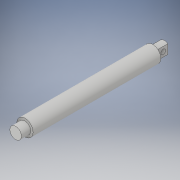
# Autodesk Inventor part: 4in stroke cylinder
Saved by Autodesk Inventor 2017 (Build 210142000, 142)
## iProperties
Created: 2017-01-19
Part Number: 4in stroke cylinder
Material: Generic
Document SubType Name: Modeling
Designer: Ben
Density: 1 g/cm^3
Appearance: Default
Author: Ben
Autodesk Inventor part; units mm, degrees
ref_plane "YZ Plane" through (0, 0, 0) normal (1, 0, 0) x (0, 1, 0)
ref_plane "XZ Plane" through (0, 0, 0) normal (0, 1, 0) x (-1, 0, 0)
ref_plane "XY Plane" through (0, 0, 0) normal (0, 0, 1) x (1, 0, 0)
sketch "Sketch1" plane through (0, 0, 0) normal (0, 0, 1) x (1, 0, 0)
  circle A0 centre (0, 0) radius 7.9375
  dimension "d0" = 15.875
  constraints: 1 centre point, 1 coincident
  measures "d0" diameter of A0
extrude "Extrusion1" add sketch "Sketch1" along normal blind 15.875
sketch "Sketch2" plane through (0, 0, 15.875) normal (0, 0, 1) x (1, 0, 0)
  circle A0 centre (0, 0) radius 11.1125
  dimension "d3" = 22.225
  constraints: 1 centre point, 1 coincident
  measures "d3" diameter of A0
extrude "Extrusion2" add sketch "Sketch2" along normal blind 174.625
sketch "Sketch3" plane through (0, 0, 190.5) normal (0, 0, 1) x (1, 0, 0)
  circle A0 centre (0, 0) radius 7.9375 projected
extrude "Extrusion3" add sketch "Sketch3" along normal blind 12.7
sketch "Sketch4" plane through (0, 0, 0) normal (0, 0, -1) x (-1, 0, 0)
  line L0 (-4.7625, 0) -> (4.7625, 0) construction
  line L1 (-4.7625, 14.2513) -> (-13.4248, 14.2513)
  line L2 (-13.4248, 14.2513) -> (-13.4248, -14.2513)
  line L3 (-13.4248, -14.2513) -> (-4.7625, -14.2513)
  line L4 (-4.7625, -14.2513) -> (-4.7625, 14.2513)
  line L5 (4.7625, 14.2513) -> (11.8991, 14.2513)
  line L6 (11.8991, 14.2513) -> (11.8991, -14.2513)
  line L7 (11.8991, -14.2513) -> (4.7625, -14.2513)
  line L8 (4.7625, -14.2513) -> (4.7625, 14.2513)
  point P0 (0, 0)
  point P1 (0, 0)
  dimension "d8" = 9.525
  constraints: 18 end point, 4 parallel, 3 horizontal, 3 midpoint, 2 perpendicular, 1 coincident, 1 point on line
  measures "d8" distance of L0.end L0.start
extrude "Extrusion4" cut sketch "Sketch4" against normal up to surface (15.875 mm away)
sketch "Sketch5" plane through (4.7625, -6.35, 0) normal (1, 0, 0) x (0, 0, -1)
  line L0 (0, 6.35) -> (-6.35, 6.35) construction
  circle A0 centre (-6.35, 6.35) radius 3.175
  dimension "d11" = 6.35
  dimension "d12" = 6.35
  constraints: 2 end point, 1 centre point, 1 coincident, 1 horizontal
  measures "d11" distance of L0.start L0.end
  measures "d12" diameter of A0
extrude "Extrusion5" cut sketch "Sketch5" against normal through all
body "Solid1"
